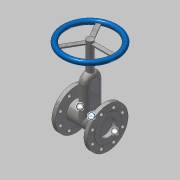
# Autodesk Inventor part: GATE VALVE FLANGED DN80
Saved by Autodesk Inventor 2017 (Build 210142000, 142)
## iProperties
Category: Piping Part
Company: Demarec
Created: 2012-12-20
Part Number: GATE VALVE FLANGED DN80
Material: S235
Document SubType Name: Modeling
Designer: Marc Crauwels
Density: 7.85 g/cm^3
Mass: 658107 g
Surface Area: 21375.3 cm^2
Volume: 83622.3 cm^3
Appearance: Steel
Catalog Web Link: http://www.pocketbrewery.com/
Author: Marc Crauwels
Title: Carbon Steel Globe Valve PN16
Comments: iPart CS GlbVlvPN16
Autodesk Inventor part; units mm, degrees
ref_plane "YZ Plane" through (0, 0, 0) normal (1, 0, 0) x (0, 1, 0)
ref_plane "XZ Plane" through (0, 0, 0) normal (0, 1, 0) x (-1, 0, 0)
ref_plane "XY Plane" through (0, 0, 0) normal (0, 0, 1) x (1, 0, 0)
sketch "Sketch1" plane through (0, 0, 0) normal (1, 0, 0) x (0, 1, 0)
  line L0 (70, 40) -> (88, 40)
  line L1 (88, 40) -> (88, 100)
  line L2 (88, 100) -> (70, 100)
  line L3 (70, 100) -> (70, 40)
  line L4 (88, 40) -> (90, 40)
  line L5 (90, 40) -> (90, 66)
  line L6 (90, 66) -> (88, 66)
  line L7 (88, 66) -> (88, 40)
  line L8 (-90, 0) -> (90, 0) construction
  line L9 (90, 0) -> (70, 0) construction
  line L10 (0, 0) -> (0, 336) construction
  line L11 (-90, 0) -> (-70, 0) construction
  line L12 (0, 0) -> (-16.6667, 0)
  line L13 (-16.6667, 0) -> (-16.6667, 336)
  line L14 (-16.6667, 336) -> (0, 336)
  line L15 (0, 336) -> (0, 0)
  line L16 (-16.6667, 326) -> (-125, 326)
  line L17 (-125, 326) -> (-125, 321)
  line L18 (-125, 321) -> (-16.6667, 321)
  line L19 (-16.6667, 321) -> (-16.6667, 326)
  circle A0 centre (-125, 323.5) radius 12.5
  dimension "Lenght" = 180
  dimension "DN" = 80
  dimension "FlgDia" = 200
  dimension "FlgThck" = 20
  dimension "GsktFace" = 132
  dimension "Height" = 336
  dimension "d48" = 16.6667
  dimension "d49" = 25
  dimension "d50" = 5
  dimension "d51" = 125
  dimension "Face" = 2
  constraints: 40 end point, 8 parallel, 7 point on line, 5 perpendicular, 4 horizontal, 2 coincident, 2 collinear, 2 midpoint, 1 centre point, 1 tangent
  measures "Lenght" distance of L8.start L8.end
  measures "DN" diameter of L0 L8
  measures "FlgDia" diameter of L2 L8
  measures "FlgThck" distance between parallel lines of L3 L5
  measures "GsktFace" diameter of L5.end L8
  measures "Height" distance of L10.start L10.end
  measures "d48" distance of L13.end L14.end
  measures "d49" diameter of A0
  measures "d50" distance of L16.end L17.end
  measures "d51" distance from line of A0.centre L10
  measures "Face" distance of L5.end L6.end
revolve "Revolution1" add sketch "Sketch1" angle 360 about axis through (0, -90, 0) along (0, 1, 0) contours L3 L2 L1 L0 | L1 L6 L5 L4
sketch "Sketch5" plane through (0, 88, 0) normal (0, 1, 0) x (1, 0, 0)
  line L0 (0, 0) -> (-30.6147, 73.9104)
  line L1 (0, 0) -> (0, 474) construction
  circle A0 centre (-30.6147, 73.9104) radius 9
  point P0 (0, 0)
  dimension "d16" = 80
  dimension "d17" = 22.5
  dimension "d18" = 18
  constraints: 4 end point, 2 coincident, 1 centre point, 1 vertical
  measures "d16" distance of L0.start L0.end
  measures "d17" angle of L1 L0
  measures "d18" diameter of A0
extrude "Extrusion2" cut sketch "Sketch5" against normal through all
pattern_circular "Circular Pattern1" count 8 over 360 about axis through (0, 89, 0) along (0, 1, 0) of "Extrusion2"
sketch "Sketch14" plane through (0, 70, 0) normal (0, -1, 0) x (-1, 0, 0)
  circle A0 centre (0, 0) radius 40 projected
  circle A1 centre (0, 0) radius 46
  dimension "d54" = 6
  constraints: 1 centre point
  measures "d54" radial gap between concentric circles of A1 A0
pattern_circular "Circular Pattern2" count 2 over 360 about axis through (-10, 0, 0) along (-1, 0, 0)
extrude "Extrusion5" add sketch "Sketch14" along normal up to surface (140 mm away) contours A0 | A1
sketch "Sketch15" plane through (0, 0, 0) normal (0, 0, 1) x (1, 0, 0)
  line L0 (46, -23) -> (-46, -23)
  line L1 (-46, -23) -> (-46, 23)
  line L2 (-46, 23) -> (46, 23)
  line L3 (46, 23) -> (46, -23)
  line L4 (-46, -23) -> (46, 23) construction
  point P0 (0, 0)
  point P1 (0, 0)
  dimension "d57" = 46
  dimension "d59" = 92
  constraints: 10 end point, 2 parallel, 1 coincident, 1 horizontal, 1 midpoint, 1 perpendicular
  measures "d57" distance of L2.end L0.start
  measures "d59" distance of L0.start L0.end
extrude "Extrusion4" add sketch "Sketch15" along normal blind 160
sketch "Sketch17" plane through (0, -23, 0) normal (0, -1, 0) x (1, 0, 0)
  line L0 (46, 160) -> (-46, 160)
  circle A0 centre (0, 160) radius 46
  line L1 (-46, 160) -> (46, 160) projected
  point P0 (0, 0)
  constraints: 2 end point, 2 midpoint, 1 collinear, 1 horizontal alignment, 2 other
extrude "Extrusion7" add sketch "Sketch17" against normal up to surface (46 mm away)
revolve "Revolution3" add sketch "Sketch1" angle 360 about axis through (0, 0, 0) along (0, 0, 1) contours L12 L13 L14 L15 | L18 A0 L16 L13 | A0 L16 L17 L18 | L18 L17 L16 A0
sketch "Sketch16" plane through (0, 0, 326) normal (0, 0, 1) x (1, 0, 0)
  line L0 (0, 0) -> (0, 112.0641) construction
  line L1 (0, 0) -> (89.1399, 51.465) construction
  line L2 (0, 0) -> (-84.4387, 48.7507) construction
  line L3 (-92.2618, 64.8144) -> (-6.547, 15.3269)
  line L4 (92.2618, 64.8144) -> (6.547, 15.3269)
  circle A0 centre (0, 0) radius 16.6667 projected
  circle A1 centre (0, 0) radius 112.7526 projected
  arc A2 (6.547, 15.3269) -> (-6.547, 15.3269) centre (0, 0) ccw
  arc A3 (92.2618, 64.8144) -> (-92.2618, 64.8144) centre (0, 0) ccw
  dimension "d61" = 120
  dimension "d62" = 60
  dimension "d63" = 10
  dimension "d64" = 10
  constraints: 10 end point, 8 point on circle, 2 centre point, 2 coincident, 2 concentric, 2 parallel, 1 vertical
  measures "d61" angle of L1 L2
  measures "d62" angle of L0 L1
  measures "d63" distance between parallel lines of L3 L2
  measures "d64" distance between parallel lines of L1 L4
extrude "Extrusion6" cut sketch "Sketch16" against normal blind 5 contours A1 L4 A0 L3 picked at (-60.6862, 52.0617)
pattern_circular "Circular Pattern3" count 3 over 360 about axis through (0, 0, 331) along (0, 0, 1) of "Extrusion6"
fillet "Fillet2" radius 23 6 edges at (-46, -23, 80) (-46, 23, 80) (0, -23, 206) (46, 23, 80) (46, -23, 80) (46, 0, 160)
equation "\"d51\" = 0.5 * WhlDia"
equation "\"d16\" = 0.5 * KDia"
equation "\"WhlDia\" = 250"
equation "\"KDia\" = 160"
body "Solid1"
